Autodesk Fusion 360 part; units mm, degrees
(part 4 of 5)
  spline S1111 degree 3 poles (22.7215, 10.5636) (22.9807, 10.5636) (23.1283, 10.5984) (23.1913, 10.6743) knots 0 0 0 0 1 1 1 1
  spline S1112 degree 3 poles (-24.4021, 10.7683) (-24.3137, 10.8038) (-23.9421, 10.9498) (-23.5763, 11.0927) knots 0 0 0 0 1 1 1 1
  spline S1113 degree 3 poles (-23.5763, 11.0927) (-22.2598, 11.6068) (-21.6203, 11.9103) (-21.579, 12.0405) knots 0 0 0 0 1 1 1 1
  spline S1114 degree 3 poles (-21.579, 12.0405) (-21.5566, 12.1111) (-21.5714, 12.2881) (-21.6118, 12.4338) knots 0 0 0 0 1 1 1 1
  spline S1115 degree 3 poles (-21.6118, 12.4338) (-21.6523, 12.5796) (-21.6856, 12.7805) (-21.6858, 12.8804) knots 0 0 0 0 1 1 1 1
  spline S1116 degree 3 poles (-21.6858, 12.8804) (-21.686, 12.9803) (-21.7458, 13.116) (-21.8186, 13.1819) knots 0 0 0 0 1 1 1 1
  spline S1117 degree 3 poles (-21.8186, 13.1819) (-21.9416, 13.2933) (-22.0025, 13.2944) (-22.6762, 13.1972) knots 0 0 0 0 1 1 1 1
  spline S1118 degree 3 poles (-22.6762, 13.1972) (-23.075, 13.1397) (-23.7635, 13.0561) (-24.2063, 13.0113) knots 0 0 0 0 1 1 1 1
  spline S1119 degree 3 poles (-24.2063, 13.0113) (-24.6491, 12.9665) (-25.0546, 12.8945) (-25.1075, 12.8511) knots 0 0 0 0 1 1 1 1
  spline S1120 degree 3 poles (-25.1075, 12.8511) (-25.2214, 12.7577) (-25.1757, 12.0662) (-25.0076, 11.3415) knots 0 0 0 0 1 1 1 1
  spline S1121 degree 3 poles (-25.0076, 11.3415) (-24.8606, 10.7078) (-24.7688, 10.6209) (-24.4021, 10.7683) knots 0 0 0 0 1 1 1 1
  spline S1122 degree 3 poles (21.2509, 11.2698) (21.326, 11.377) (21.3366, 11.4739) (21.2907, 11.634) knots 0 0 0 0 1 1 1 1
  spline S1123 degree 3 poles (21.2907, 11.634) (21.1709, 12.0516) (21.2089, 12.044) (18.9436, 12.1086) knots 0 0 0 0 1 1 1 1
  spline S1124 degree 3 poles (18.9436, 12.1086) (17.0607, 12.1623) (16.8438, 12.157) (16.7302, 12.0542) knots 0 0 0 0 1 1 1 1
  spline S1125 degree 3 poles (16.7302, 12.0542) (16.6337, 11.9669) (16.6147, 11.8816) (16.6491, 11.6895) knots 0 0 0 0 1 1 1 1
  spline S1126 degree 3 poles (16.6491, 11.6895) (16.7375, 11.1953) (16.7258, 11.1985) (18.4885, 11.1761) knots 0 0 0 0 1 1 1 1
  spline S1127 degree 3 poles (18.4885, 11.1761) (19.3591, 11.165) (20.3138, 11.1487) (20.61, 11.1398) knots 0 0 0 0 1 1 1 1
  spline S1128 degree 3 poles (20.61, 11.1398) (21.0869, 11.1255) (21.1603, 11.1404) (21.2509, 11.2698) knots 0 0 0 0 1 1 1 1
  spline S1129 degree 3 poles (-19.2079, 11.7134) (-18.8576, 11.9992) (-18.3505, 12.4375) (-18.0809, 12.6873) knots 0 0 0 0 1 1 1 1
  spline S1130 degree 3 poles (-18.0809, 12.6873) (-17.6144, 13.1198) (-17.5967, 13.1475) (-17.7119, 13.2662) knots 0 0 0 0 1 1 1 1
  spline S1131 degree 3 poles (-17.7119, 13.2662) (-17.8279, 13.3856) (-17.8483, 13.3846) (-18.202, 13.2406) knots 0 0 0 0 1 1 1 1
  spline S1132 degree 3 poles (-18.202, 13.2406) (-19.0738, 12.8857) (-20.2187, 12.4538) (-20.2877, 12.4538) knots 0 0 0 0 1 1 1 1
  spline S1133 degree 3 poles (-20.2877, 12.4538) (-20.3288, 12.4538) (-20.4422, 12.374) (-20.5396, 12.2766) knots 0 0 0 0 1 1 1 1
  line L139 (-20.5396, 12.2766) -> (-20.7168, 12.0994)
  line L140 (-20.7168, 12.0994) -> (-20.5267, 11.769)
  spline S1134 degree 3 poles (-20.5267, 11.769) (-20.2684, 11.3201) (-20.1493, 11.1937) (-19.9846, 11.1937) knots 0 0 0 0 1 1 1 1
  spline S1135 degree 3 poles (-19.9846, 11.1937) (-19.9078, 11.1937) (-19.5583, 11.4275) (-19.2079, 11.7134) knots 0 0 0 0 1 1 1 1
  spline S1136 degree 3 poles (-13.2368, 11.7436) (-12.6043, 12.2729) (-12.0764, 12.8629) (-12.1241, 12.9872) knots 0 0 0 0 1 1 1 1
  spline S1137 degree 3 poles (-12.1241, 12.9872) (-12.1469, 13.0466) (-12.1656, 13.1242) (-12.1656, 13.1595) knots 0 0 0 0 1 1 1 1
  spline S1138 degree 3 poles (-12.1656, 13.1595) (-12.1656, 13.1949) (-12.1975, 13.2238) (-12.2366, 13.2238) knots 0 0 0 0 1 1 1 1
  spline S1139 degree 3 poles (-12.2366, 13.2238) (-12.2756, 13.2238) (-12.7001, 13.4012) (-13.1798, 13.6181) knots 0 0 0 0 1 1 1 1
  spline S1140 degree 3 poles (-13.1798, 13.6181) (-14.0327, 14.0036) (-14.0561, 14.0097) (-14.2327, 13.894) knots 0 0 0 0 1 1 1 1
  spline S1141 degree 3 poles (-14.2327, 13.894) (-14.332, 13.8289) (-14.4315, 13.7282) (-14.4538, 13.6701) knots 0 0 0 0 1 1 1 1
  spline S1142 degree 3 poles (-14.4538, 13.6701) (-14.512, 13.5184) (-13.9849, 11.5956) (-13.8565, 11.4912) knots 0 0 0 0 1 1 1 1
  spline S1143 degree 3 poles (-13.8565, 11.4912) (-13.6999, 11.3638) (-13.6817, 11.3712) (-13.2368, 11.7436) knots 0 0 0 0 1 1 1 1
  spline S1144 degree 3 poles (-8.9533, 13.0095) (-8.8858, 13.0457) (-8.7742, 13.2) (-8.7055, 13.3525) knots 0 0 0 0 1 1 1 1
  spline S1145 degree 3 poles (-8.7055, 13.3525) (-8.4998, 13.8087) (-8.5846, 13.8736) (-9.5179, 13.9744) knots 0 0 0 0 1 1 1 1
  line L141 (-9.5179, 13.9744) -> (-10.3105, 14.06)
  line L142 (-10.3105, 14.06) -> (-10.468, 13.883)
  spline S1146 degree 3 poles (-10.468, 13.883) (-10.7752, 13.5378) (-10.6837, 13.4311) (-9.8554, 13.1682) knots 0 0 0 0 1 1 1 1
  spline S1147 degree 3 poles (-9.8554, 13.1682) (-9.0718, 12.9194) (-9.1093, 12.926) (-8.9533, 13.0095) knots 0 0 0 0 1 1 1 1
  spline S1148 degree 3 poles (-18.991, 13.7481) (-18.7215, 13.8542) (-18.2394, 14.0518) (-17.9197, 14.1873) knots 0 0 0 0 1 1 1 1
  spline S1149 degree 3 poles (-17.9197, 14.1873) (-17.3857, 14.4137) (-17.3402, 14.4485) (-17.3597, 14.6163) knots 0 0 0 0 1 1 1 1
  line L143 (-17.3597, 14.6163) -> (-17.3809, 14.7989)
  line L144 (-17.3809, 14.7989) -> (-19.026, 14.8367)
  spline S1150 degree 3 poles (-19.026, 14.8367) (-21.0331, 14.8829) (-20.9284, 14.9282) (-20.9731, 13.9937) knots 0 0 0 0 1 1 1 1
  spline S1151 degree 3 poles (-20.9731, 13.9937) (-20.9985, 13.4622) (-20.9838, 13.3373) (-20.8825, 13.2253) knots 0 0 0 0 1 1 1 1
  spline S1152 degree 3 poles (-20.8825, 13.2253) (-20.7638, 13.0942) (-20.749, 13.0961) (-20.1212, 13.3234) knots 0 0 0 0 1 1 1 1
  spline S1153 degree 3 poles (-20.1212, 13.3234) (-19.7691, 13.4509) (-19.2605, 13.642) (-18.991, 13.7481) knots 0 0 0 0 1 1 1 1
  spline S1154 degree 3 poles (-23.3146, 13.8917) (-22.5289, 13.9927) (-21.893, 14.1075) (-21.8429, 14.1575) knots 0 0 0 0 1 1 1 1
  spline S1155 degree 3 poles (-21.8429, 14.1575) (-21.7944, 14.2058) (-21.7099, 14.4959) (-21.6552, 14.8022) knots 0 0 0 0 1 1 1 1
  spline S1156 degree 3 poles (-21.6552, 14.8022) (-21.6005, 15.1084) (-21.5059, 15.4981) (-21.4449, 15.6681) knots 0 0 0 0 1 1 1 1
  spline S1157 degree 3 poles (-21.4449, 15.6681) (-21.384, 15.8382) (-21.3519, 16.0334) (-21.3737, 16.1019) knots 0 0 0 0 1 1 1 1
  spline S1158 degree 3 poles (-21.3737, 16.1019) (-21.396, 16.1723) (-21.5793, 16.2891) (-21.7947, 16.3703) knots 0 0 0 0 1 1 1 1
  spline S1159 degree 3 poles (-21.7947, 16.3703) (-22.0045, 16.4493) (-22.3573, 16.5815) (-22.5787, 16.664) knots 0 0 0 0 1 1 1 1
  spline S1160 degree 3 poles (-22.5787, 16.664) (-22.8001, 16.7464) (-23.2138, 16.9206) (-23.4981, 17.0509) knots 0 0 0 0 1 1 1 1
  spline S1161 degree 3 poles (-23.4981, 17.0509) (-23.9693, 17.267) (-24.0287, 17.279) (-24.1702, 17.1862) knots 0 0 0 0 1 1 1 1
  spline S1162 degree 3 poles (-24.1702, 17.1862) (-24.5551, 16.9341) (-25.2902, 14.1127) (-25.0473, 13.82) knots 0 0 0 0 1 1 1 1
  spline S1163 degree 3 poles (-25.0473, 13.82) (-24.9336, 13.683) (-24.9403, 13.6827) (-23.3146, 13.8917) knots 0 0 0 0 1 1 1 1
  spline S1164 degree 3 poles (-11.5027, 13.8277) (-11.4398, 13.8518) (-11.2771, 14.0925) (-11.1411, 14.3625) knots 0 0 0 0 1 1 1 1
  spline S1165 degree 3 poles (-11.1411, 14.3625) (-10.902, 14.8374) (-10.8981, 14.8575) (-11.0222, 14.9768) knots 0 0 0 0 1 1 1 1
  spline S1166 degree 3 poles (-11.0222, 14.9768) (-11.1429, 15.0929) (-11.2111, 15.0941) (-12.1656, 14.9984) knots 0 0 0 0 1 1 1 1
  spline S1167 degree 3 poles (-12.1656, 14.9984) (-13.3577, 14.8788) (-13.3556, 14.8794) (-13.3556, 14.6979) knots 0 0 0 0 1 1 1 1
  spline S1168 degree 3 poles (-13.3556, 14.6979) (-13.3556, 14.5391) (-13.2065, 14.4507) (-12.2706, 14.0546) knots 0 0 0 0 1 1 1 1
  spline S1169 degree 3 poles (-12.2706, 14.0546) (-11.5304, 13.7413) (-11.6419, 13.7743) (-11.5027, 13.8277) knots 0 0 0 0 1 1 1 1
  spline S1170 degree 3 poles (-15.122, 14.2422) (-14.6101, 14.4561) (-14.2657, 14.9516) (-14.2657, 15.4741) knots 0 0 0 0 1 1 1 1
  spline S1171 degree 3 poles (-14.2657, 15.4741) (-14.2657, 15.8959) (-14.4671, 16.094) (-14.8959, 16.094) knots 0 0 0 0 1 1 1 1
  spline S1172 degree 3 poles (-14.8959, 16.094) (-15.8095, 16.094) (-16.5832, 14.8175) (-15.9994, 14.2736) knots 0 0 0 0 1 1 1 1
  spline S1173 degree 3 poles (-15.9994, 14.2736) (-15.8183, 14.1049) (-15.4797, 14.0927) (-15.122, 14.2422) knots 0 0 0 0 1 1 1 1
  spline S1174 degree 3 poles (-8.003, 14.785) (-7.8424, 15.0302) (-7.341, 16.6099) (-7.3194, 16.939) knots 0 0 0 0 1 1 1 1
  spline S1175 degree 3 poles (-7.3194, 16.939) (-7.2863, 17.4417) (-7.3904, 17.4406) (-8.5646, 16.9264) knots 0 0 0 0 1 1 1 1
  spline S1176 degree 3 poles (-8.5646, 16.9264) (-9.1332, 16.6774) (-9.6221, 16.4276) (-9.6509, 16.3713) knots 0 0 0 0 1 1 1 1
  spline S1177 degree 3 poles (-9.6509, 16.3713) (-9.6797, 16.3151) (-9.7716, 15.9734) (-9.8551, 15.6122) knots 0 0 0 0 1 1 1 1
  spline S1178 degree 3 poles (-9.8551, 15.6122) (-10.0402, 14.8114) (-10.0253, 14.7874) (-9.2924, 14.7025) knots 0 0 0 0 1 1 1 1
  spline S1179 degree 3 poles (-9.2924, 14.7025) (-8.3312, 14.5912) (-8.1212, 14.6046) (-8.003, 14.785) knots 0 0 0 0 1 1 1 1
  spline S1180 degree 3 poles (-17.7099, 15.6179) (-17.5251, 15.8028) (-17.6358, 15.9384) (-18.3085, 16.3507) knots 0 0 0 0 1 1 1 1
  spline S1181 degree 3 poles (-18.3085, 16.3507) (-18.6839, 16.5809) (-19.1537, 16.8723) (-19.3526, 16.9984) knots 0 0 0 0 1 1 1 1
  spline S1182 degree 3 poles (-19.3526, 16.9984) (-19.6303, 17.1744) (-19.7429, 17.2116) (-19.8376, 17.1586) knots 0 0 0 0 1 1 1 1
  spline S1183 degree 3 poles (-19.8376, 17.1586) (-19.9055, 17.1206) (-20.0957, 16.8262) (-20.2603, 16.5042) knots 0 0 0 0 1 1 1 1
  spline S1184 degree 3 poles (-20.2603, 16.5042) (-20.6962, 15.6518) (-20.6935, 15.6494) (-19.2276, 15.6013) knots 0 0 0 0 1 1 1 1
  spline S1185 degree 3 poles (-19.2276, 15.6013) (-18.597, 15.5806) (-18.0164, 15.557) (-17.9374, 15.5488) knots 0 0 0 0 1 1 1 1
  spline S1186 degree 3 poles (-17.9374, 15.5488) (-17.8585, 15.5406) (-17.7561, 15.5717) (-17.7099, 15.6179) knots 0 0 0 0 1 1 1 1
  spline S1187 degree 3 poles (-11.1991, 15.8565) (-10.6041, 15.9191) (-10.4912, 16.0246) (-10.4685, 16.5393) knots 0 0 0 0 1 1 1 1
  spline S1188 degree 3 poles (-10.4685, 16.5393) (-10.4402, 17.1834) (-10.5209, 17.1892) (-11.4906, 16.6128) knots 0 0 0 0 1 1 1 1
  spline S1189 degree 3 poles (-11.4906, 16.6128) (-12.1123, 16.2431) (-12.3045, 16.0946) (-12.305, 15.9831) knots 0 0 0 0 1 1 1 1
  spline S1190 degree 3 poles (-12.305, 15.9831) (-12.3058, 15.7689) (-12.2332, 15.7288) (-11.921, 15.7717) knots 0 0 0 0 1 1 1 1
  spline S1191 degree 3 poles (-11.921, 15.7717) (-11.7668, 15.7928) (-11.4419, 15.831) (-11.1991, 15.8565) knots 0 0 0 0 1 1 1 1
  spline S1192 degree 3 poles (-29.4487, 16.0958) (-29.2413, 16.1353) (-28.2608, 16.2435) (-27.2697, 16.3363) knots 0 0 0 0 1 1 1 1
  spline S1193 degree 3 poles (-27.2697, 16.3363) (-26.2787, 16.429) (-25.4399, 16.5221) (-25.4057, 16.5432) knots 0 0 0 0 1 1 1 1
  spline S1194 degree 3 poles (-25.4057, 16.5432) (-25.3716, 16.5643) (-25.2714, 16.7633) (-25.1832, 16.9853) knots 0 0 0 0 1 1 1 1
  spline S1195 degree 3 poles (-25.1832, 16.9853) (-24.9857, 17.4823) (-24.5021, 18.4625) (-24.2095, 18.9587) knots 0 0 0 0 1 1 1 1
  spline S1196 degree 3 poles (-24.2095, 18.9587) (-24.0275, 19.2675) (-24.0058, 19.3479) (-24.079, 19.444) knots 0 0 0 0 1 1 1 1
  spline S1197 degree 3 poles (-24.079, 19.444) (-24.1272, 19.5074) (-24.1706, 19.5673) (-24.1754, 19.5772) knots 0 0 0 0 1 1 1 1
  spline S1198 degree 3 poles (-24.1754, 19.5772) (-24.192, 19.6118) (-26.0679, 19.3801) (-26.9015, 19.2405) knots 0 0 0 0 1 1 1 1
  spline S1199 degree 3 poles (-26.9015, 19.2405) (-27.3635, 19.1631) (-27.932, 19.0374) (-28.1647, 18.9611) knots 0 0 0 0 1 1 1 1
  spline S1200 degree 3 poles (-28.1647, 18.9611) (-28.5842, 18.8235) (-28.5912, 18.8168) (-28.9823, 18.1757) knots 0 0 0 0 1 1 1 1
  spline S1201 degree 3 poles (-28.9823, 18.1757) (-29.1993, 17.82) (-29.5234, 17.2641) (-29.7025, 16.9402) knots 0 0 0 0 1 1 1 1
  spline S1202 degree 3 poles (-29.7025, 16.9402) (-29.9932, 16.4146) (-30.0188, 16.3337) (-29.9406, 16.1876) knots 0 0 0 0 1 1 1 1
  spline S1203 degree 3 poles (-29.9406, 16.1876) (-29.8924, 16.0976) (-29.8469, 16.024) (-29.8394, 16.024) knots 0 0 0 0 1 1 1 1
  spline S1204 degree 3 poles (-29.8394, 16.024) (-29.8319, 16.024) (-29.6561, 16.0563) (-29.4487, 16.0958) knots 0 0 0 0 1 1 1 1
  spline S1205 degree 3 poles (-16.2395, 16.4188) (-16.2187, 16.5646) (-16.4568, 17.3401) (-16.9745, 18.8132) knots 0 0 0 0 1 1 1 1
  spline S1206 degree 3 poles (-16.9745, 18.8132) (-17.2943, 19.723) (-17.3662, 19.7643) (-17.906, 19.3491) knots 0 0 0 0 1 1 1 1
  spline S1207 degree 3 poles (-17.906, 19.3491) (-18.4508, 18.93) (-19.236, 18.1166) (-19.236, 17.9714) knots 0 0 0 0 1 1 1 1
  spline S1208 degree 3 poles (-19.236, 17.9714) (-19.236, 17.848) (-18.823, 17.5592) (-17.3849, 16.6773) knots 0 0 0 0 1 1 1 1
  spline S1209 degree 3 poles (-17.3849, 16.6773) (-16.6183, 16.2071) (-16.2805, 16.1309) (-16.2395, 16.4188) knots 0 0 0 0 1 1 1 1
  spline S1210 degree 3 poles (24.6841, 16.7418) (24.7472, 16.8421) (24.6348, 17.1146) (24.0681, 18.2358) knots 0 0 0 0 1 1 1 1
  spline S1211 degree 3 poles (24.0681, 18.2358) (23.6075, 19.147) (23.3258, 19.6277) (23.2283, 19.6685) knots 0 0 0 0 1 1 1 1
  spline S1212 degree 3 poles (23.2283, 19.6685) (23.1476, 19.7022) (22.4538, 19.7782) (21.6865, 19.8372) knots 0 0 0 0 1 1 1 1
  spline S1213 degree 3 poles (21.6865, 19.8372) (20.7303, 19.9108) (20.2419, 19.977) (20.134, 20.0476) knots 0 0 0 0 1 1 1 1
  spline S1214 degree 3 poles (20.134, 20.0476) (20.0474, 20.1044) (19.797, 20.4587) (19.5775, 20.835) knots 0 0 0 0 1 1 1 1
  spline S1215 degree 3 poles (19.5775, 20.835) (19.358, 21.2114) (19.0588, 21.6802) (18.9126, 21.8768) knots 0 0 0 0 1 1 1 1
  line L145 (18.9126, 21.8768) -> (18.6469, 22.2344)
  line L146 (18.6469, 22.2344) -> (17.294, 22.3167)
  spline S1216 degree 3 poles (17.294, 22.3167) (16.55, 22.362) (15.8373, 22.412) (15.7104, 22.4278) knots 0 0 0 0 1 1 1 1
  spline S1217 degree 3 poles (15.7104, 22.4278) (15.5213, 22.4514) (15.4661, 22.427) (15.4048, 22.2924) knots 0 0 0 0 1 1 1 1
  spline S1218 degree 3 poles (15.4048, 22.2924) (15.3433, 22.1575) (15.3768, 22.007) (15.5924, 21.4507) knots 0 0 0 0 1 1 1 1
  line L147 (15.5924, 21.4507) -> (15.8549, 20.7732)
  line L148 (15.8549, 20.7732) -> (15.6497, 20.4812)
  line L149 (15.6497, 20.4812) -> (15.4444, 20.1892)
  line L150 (15.4444, 20.1892) -> (14.5027, 20.2093)
  spline S1219 degree 3 poles (14.5027, 20.2093) (13.9848, 20.2204) (13.2933, 20.2428) (12.966, 20.2592) knots 0 0 0 0 1 1 1 1
  spline S1220 degree 3 poles (12.966, 20.2592) (12.6387, 20.2755) (11.5034, 20.3093) (10.4432, 20.3342) knots 0 0 0 0 1 1 1 1
  spline S1221 degree 3 poles (10.4432, 20.3342) (8.7029, 20.375) (8.5061, 20.3681) (8.4196, 20.2639) knots 0 0 0 0 1 1 1 1
  spline S1222 degree 3 poles (8.4196, 20.2639) (8.3377, 20.1652) (8.3576, 19.9424) (8.556, 18.7337) knots 0 0 0 0 1 1 1 1
  spline S1223 degree 3 poles (8.556, 18.7337) (8.711, 17.7902) (8.8254, 17.2814) (8.8995, 17.206) knots 0 0 0 0 1 1 1 1
  spline S1224 degree 3 poles (8.8995, 17.206) (8.9972, 17.1068) (9.5698, 17.0787) (13.596, 16.9752) knots 0 0 0 0 1 1 1 1
  spline S1225 degree 3 poles (13.596, 16.9752) (18.7286, 16.8432) (19.6049, 16.8128) (21.8565, 16.6884) knots 0 0 0 0 1 1 1 1
  spline S1226 degree 3 poles (21.8565, 16.6884) (23.9806, 16.5711) (24.5839, 16.5825) (24.6841, 16.7418) knots 0 0 0 0 1 1 1 1
  spline S1227 degree 3 poles (-11.963, 17.225) (-11.6316, 17.4236) (-11.1758, 17.7107) (-10.9501, 17.863) knots 0 0 0 0 1 1 1 1
  spline S1228 degree 3 poles (-10.9501, 17.863) (-10.5619, 18.1251) (-10.5418, 18.1526) (-10.5777, 18.3738) knots 0 0 0 0 1 1 1 1
  spline S1229 degree 3 poles (-10.5777, 18.3738) (-10.6459, 18.794) (-10.9302, 19.2768) (-11.123, 19.2999) knots 0 0 0 0 1 1 1 1
  spline S1230 degree 3 poles (-11.123, 19.2999) (-11.2688, 19.3174) (-11.3514, 19.2395) (-11.6426, 18.8099) knots 0 0 0 0 1 1 1 1
  spline S1231 degree 3 poles (-11.6426, 18.8099) (-11.833, 18.529) (-12.1895, 18.0229) (-12.4348, 17.6853) knots 0 0 0 0 1 1 1 1
  spline S1232 degree 3 poles (-12.4348, 17.6853) (-12.8031, 17.1783) (-12.8657, 17.0535) (-12.7946, 16.9678) knots 0 0 0 0 1 1 1 1
  spline S1233 degree 3 poles (-12.7946, 16.9678) (-12.7472, 16.9107) (-12.6763, 16.864) (-12.637, 16.864) knots 0 0 0 0 1 1 1 1
  spline S1234 degree 3 poles (-12.637, 16.864) (-12.5977, 16.864) (-12.2944, 17.0265) (-11.963, 17.225) knots 0 0 0 0 1 1 1 1
  spline S1235 degree 3 poles (-20.8903, 17.0639) (-20.8256, 17.1354) (-20.7917, 17.2431) (-20.8148, 17.3034) knots 0 0 0 0 1 1 1 1
  spline S1236 degree 3 poles (-20.8148, 17.3034) (-20.8533, 17.4038) (-22.872, 18.7732) (-23.1241, 18.8699) knots 0 0 0 0 1 1 1 1
  spline S1237 degree 3 poles (-23.1241, 18.8699) (-23.3444, 18.9545) (-23.7875, 18.3407) (-23.6899, 18.0863) knots 0 0 0 0 1 1 1 1
  spline S1238 degree 3 poles (-23.6899, 18.0863) (-23.6666, 18.0255) (-23.4346, 17.8783) (-23.1744, 17.7589) knots 0 0 0 0 1 1 1 1
  spline S1239 degree 3 poles (-23.1744, 17.7589) (-22.5961, 17.4938) (-21.1899, 16.9406) (-21.0845, 16.9368) knots 0 0 0 0 1 1 1 1
  spline S1240 degree 3 poles (-21.0845, 16.9368) (-21.0423, 16.9353) (-20.9549, 16.9925) (-20.8903, 17.0639) knots 0 0 0 0 1 1 1 1
  spline S1241 degree 3 poles (-1.9745, 17.2186) (-1.9197, 17.264) (-1.876, 17.729) (-1.8449, 18.5982) knots 0 0 0 0 1 1 1 1
  spline S1242 degree 3 poles (-1.8449, 18.5982) (-1.7806, 20.3917) (-1.6759, 22.7737) (-1.624, 23.6226) knots 0 0 0 0 1 1 1 1
  spline S1243 degree 3 poles (-1.624, 23.6226) (-1.5882, 24.2076) (-1.5991, 24.3408) (-1.6891, 24.4155) knots 0 0 0 0 1 1 1 1
  spline S1244 degree 3 poles (-1.6891, 24.4155) (-1.8113, 24.5169) (-3.3464, 24.5276) (-6.4842, 24.4489) knots 0 0 0 0 1 1 1 1
  spline S1245 degree 3 poles (-6.4842, 24.4489) (-8.3278, 24.4026) (-8.3283, 24.4025) (-8.4027, 24.2393) knots 0 0 0 0 1 1 1 1
  spline S1246 degree 3 poles (-8.4027, 24.2393) (-8.4687, 24.0945) (-8.4379, 24.0343) (-8.1304, 23.7077) knots 0 0 0 0 1 1 1 1
  spline S1247 degree 3 poles (-8.1304, 23.7077) (-6.8687, 22.3676) (-6.2732, 20.5027) (-6.3844, 18.2404) knots 0 0 0 0 1 1 1 1
  spline S1248 degree 3 poles (-6.3844, 18.2404) (-6.4135, 17.6483) (-6.4058, 17.24) (-6.3646, 17.1903) knots 0 0 0 0 1 1 1 1
  spline S1249 degree 3 poles (-6.3646, 17.1903) (-6.2792, 17.0872) (-2.1003, 17.1142) (-1.9745, 17.2186) knots 0 0 0 0 1 1 1 1
  spline S1250 degree 3 poles (7.9228, 17.1756) (8.0336, 17.3091) (7.9974, 17.6663) (7.7218, 19.1614) knots 0 0 0 0 1 1 1 1
  spline S1251 degree 3 poles (7.7218, 19.1614) (7.6131, 19.7512) (7.487, 20.2709) (7.4414, 20.3165) knots 0 0 0 0 1 1 1 1
  spline S1252 degree 3 poles (7.4414, 20.3165) (7.3827, 20.3753) (6.7665, 20.406) (5.3145, 20.4227) knots 0 0 0 0 1 1 1 1
  line L151 (5.3145, 20.4227) -> (3.2704, 20.4461)
  line L152 (3.2704, 20.4461) -> (3.048, 20.6589)
  spline S1253 degree 3 poles (3.048, 20.6589) (2.8474, 20.8509) (2.8214, 20.924) (2.7826, 21.4055) knots 0 0 0 0 1 1 1 1
  spline S1254 degree 3 poles (2.7826, 21.4055) (2.662, 22.8997) (2.5206, 24.1965) (2.4629, 24.337) knots 0 0 0 0 1 1 1 1
  spline S1255 degree 3 poles (2.4629, 24.337) (2.3987, 24.4936) (2.3893, 24.4945) (0.8653, 24.4945) knots 0 0 0 0 1 1 1 1
  spline S1256 degree 3 poles (0.8653, 24.4945) (-0.4157, 24.4945) (-0.6821, 24.4771) (-0.7554, 24.3889) knots 0 0 0 0 1 1 1 1
  spline S1257 degree 3 poles (-0.7554, 24.3889) (-0.8521, 24.2723) (-0.9043, 23.4082) (-1.0395, 19.6829) knots 0 0 0 0 1 1 1 1
  spline S1258 degree 3 poles (-1.0395, 19.6829) (-1.107, 17.8242) (-1.1064, 17.3352) (-1.0364, 17.2509) knots 0 0 0 0 1 1 1 1
  spline S1259 degree 3 poles (-1.0364, 17.2509) (-0.961, 17.16) (-0.4774, 17.1428) (2.4559, 17.1272) knots 0 0 0 0 1 1 1 1
  spline S1260 degree 3 poles (2.4559, 17.1272) (4.3284, 17.1172) (6.3041, 17.0994) (6.8462, 17.0876) knots 0 0 0 0 1 1 1 1
  spline S1261 degree 3 poles (6.8462, 17.0876) (7.6728, 17.0696) (7.8466, 17.0838) (7.9228, 17.1756) knots 0 0 0 0 1 1 1 1
  spline S1262 degree 3 poles (-8.3794, 17.8468) (-7.0575, 18.4432) (-7.1146, 18.394) (-7.1395, 18.9154) knots 0 0 0 0 1 1 1 1
  spline S1263 degree 3 poles (-7.1395, 18.9154) (-7.1578, 19.2983) (-7.1779, 19.3517) (-7.3109, 19.3706) knots 0 0 0 0 1 1 1 1
  spline S1264 degree 3 poles (-7.3109, 19.3706) (-7.483, 19.3952) (-9.6454, 17.83) (-9.6454, 17.6809) knots 0 0 0 0 1 1 1 1
  spline S1265 degree 3 poles (-9.6454, 17.6809) (-9.6454, 17.5701) (-9.5041, 17.4241) (-9.3968, 17.4241) knots 0 0 0 0 1 1 1 1
  spline S1266 degree 3 poles (-9.3968, 17.4241) (-9.3525, 17.4241) (-8.8947, 17.6143) (-8.3794, 17.8468) knots 0 0 0 0 1 1 1 1
  spline S1267 degree 3 poles (-15.3671, 18.053) (-15.3369, 18.2641) (-15.3209, 18.8907) (-15.3315, 19.4455) knots 0 0 0 0 1 1 1 1
  spline S1268 degree 3 poles (-15.3315, 19.4455) (-15.3551, 20.6788) (-15.3656, 20.6931) (-16.0392, 20.4068) knots 0 0 0 0 1 1 1 1
  spline S1269 degree 3 poles (-16.0392, 20.4068) (-16.29, 20.3002) (-16.5129, 20.1668) (-16.5346, 20.1103) knots 0 0 0 0 1 1 1 1
  spline S1270 degree 3 poles (-16.5346, 20.1103) (-16.5563, 20.0538) (-16.3933, 19.4725) (-16.1724, 18.8184) knots 0 0 0 0 1 1 1 1
  spline S1271 degree 3 poles (-16.1724, 18.8184) (-15.7888, 17.6826) (-15.763, 17.6302) (-15.5964, 17.6492) knots 0 0 0 0 1 1 1 1
  spline S1272 degree 3 poles (-15.5964, 17.6492) (-15.4421, 17.6668) (-15.4157, 17.7133) (-15.3671, 18.053) knots 0 0 0 0 1 1 1 1
  spline S1273 degree 3 poles (-19.9804, 18.3806) (-19.8405, 18.5602) (-19.726, 18.7507) (-19.726, 18.804) knots 0 0 0 0 1 1 1 1
  spline S1274 degree 3 poles (-19.726, 18.804) (-19.726, 18.8573) (-19.9944, 19.2023) (-20.3223, 19.5707) knots 0 0 0 0 1 1 1 1
  spline S1275 degree 3 poles (-20.3223, 19.5707) (-20.6503, 19.939) (-21.0362, 20.3929) (-21.1799, 20.5794) knots 0 0 0 0 1 1 1 1
  spline S1276 degree 3 poles (-21.1799, 20.5794) (-21.5341, 21.039) (-21.6932, 21.0349) (-22.1105, 20.5559) knots 0 0 0 0 1 1 1 1
  spline S1277 degree 3 poles (-22.1105, 20.5559) (-22.6039, 19.9894) (-22.7587, 19.7538) (-22.7141, 19.6374) knots 0 0 0 0 1 1 1 1
  spline S1278 degree 3 poles (-22.7141, 19.6374) (-22.6624, 19.5027) (-20.501, 18.0579) (-20.3479, 18.0557) knots 0 0 0 0 1 1 1 1
  spline S1279 degree 3 poles (-20.3479, 18.0557) (-20.2857, 18.0548) (-20.1203, 18.201) (-19.9804, 18.3806) knots 0 0 0 0 1 1 1 1
  spline S1280 degree 3 poles (-13.8919, 18.9349) (-13.7055, 19.3937) (-13.4904, 19.9226) (-13.4138, 20.11) knots 0 0 0 0 1 1 1 1
  spline S1281 degree 3 poles (-13.4138, 20.11) (-13.1823, 20.6768) (-13.3092, 20.8511) (-13.9548, 20.8533) knots 0 0 0 0 1 1 1 1
  spline S1282 degree 3 poles (-13.9548, 20.8533) (-14.4887, 20.8551) (-14.5056, 20.8149) (-14.5498, 19.4425) knots 0 0 0 0 1 1 1 1
  spline S1283 degree 3 poles (-14.5498, 19.4425) (-14.583, 18.4103) (-14.573, 18.2159) (-14.4826, 18.1407) knots 0 0 0 0 1 1 1 1
  spline S1284 degree 3 poles (-14.4826, 18.1407) (-14.4242, 18.092) (-14.3436, 18.0631) (-14.3035, 18.0764) knots 0 0 0 0 1 1 1 1
  spline S1285 degree 3 poles (-14.3035, 18.0764) (-14.2635, 18.0896) (-14.0782, 18.476) (-13.8919, 18.9349) knots 0 0 0 0 1 1 1 1
  spline S1286 degree 3 poles (-12.3167, 19.2004) (-11.7607, 20.0152) (-11.7206, 20.1966) (-12.0622, 20.3522) knots 0 0 0 0 1 1 1 1
  spline S1287 degree 3 poles (-12.0622, 20.3522) (-12.4177, 20.5142) (-12.4624, 20.4628) (-12.8606, 19.432) knots 0 0 0 0 1 1 1 1
  spline S1288 degree 3 poles (-12.8606, 19.432) (-13.1686, 18.635) (-13.1918, 18.5374) (-13.0871, 18.4765) knots 0 0 0 0 1 1 1 1
  spline S1289 degree 3 poles (-13.0871, 18.4765) (-13.0231, 18.4392) (-12.9391, 18.4173) (-12.9006, 18.4279) knots 0 0 0 0 1 1 1 1
  spline S1290 degree 3 poles (-12.9006, 18.4279) (-12.8621, 18.4385) (-12.5993, 18.7861) (-12.3167, 19.2004) knots 0 0 0 0 1 1 1 1
  spline S1291 degree 3 poles (-8.7354, 19.4121) (-8.2541, 19.7731) (-7.7347, 20.1784) (-7.5812, 20.3126) knots 0 0 0 0 1 1 1 1
  line L153 (-7.5812, 20.3126) -> (-7.3021, 20.5567)
  line L154 (-7.3021, 20.5567) -> (-7.4675, 21.073)
  spline S1292 degree 3 poles (-7.4675, 21.073) (-7.7543, 21.9682) (-8.1644, 22.664) (-8.793, 23.3219) knots 0 0 0 0 1 1 1 1
  spline S1293 degree 3 poles (-8.793, 23.3219) (-9.0651, 23.6067) (-9.3183, 23.6618) (-9.437, 23.4619) knots 0 0 0 0 1 1 1 1
  spline S1294 degree 3 poles (-9.437, 23.4619) (-9.477, 23.3946) (-9.8553, 22.7592) (-10.2776, 22.0501) knots 0 0 0 0 1 1 1 1
  spline S1295 degree 3 poles (-10.2776, 22.0501) (-10.7, 21.3409) (-11.0455, 20.7206) (-11.0455, 20.6715) knots 0 0 0 0 1 1 1 1
  spline S1296 degree 3 poles (-11.0455, 20.6715) (-11.0455, 20.6225) (-10.8868, 20.401) (-10.6927, 20.1793) knots 0 0 0 0 1 1 1 1
  spline S1297 degree 3 poles (-10.6927, 20.1793) (-10.4987, 19.9576) (-10.2388, 19.5636) (-10.1152, 19.3038) knots 0 0 0 0 1 1 1 1
  spline S1298 degree 3 poles (-10.1152, 19.3038) (-9.9211, 18.8958) (-9.8416, 18.8044) (-9.6454, 18.763) knots 0 0 0 0 1 1 1 1
  spline S1299 degree 3 poles (-9.6454, 18.763) (-9.6262, 18.7589) (-9.2166, 19.051) (-8.7354, 19.4121) knots 0 0 0 0 1 1 1 1
  spline S1300 degree 3 poles (-18.6774, 19.7262) (-18.5, 19.8758) (-18.1042, 20.1617) (-17.7979, 20.3616) knots 0 0 0 0 1 1 1 1
  spline S1301 degree 3 poles (-17.7979, 20.3616) (-17.4915, 20.5615) (-17.2154, 20.7704) (-17.1842, 20.8259) knots 0 0 0 0 1 1 1 1
  spline S1302 degree 3 poles (-17.1842, 20.8259) (-17.1495, 20.8878) (-17.2127, 21.1625) (-17.3482, 21.538) knots 0 0 0 0 1 1 1 1
  spline S1303 degree 3 poles (-17.3482, 21.538) (-18.0947, 23.607) (-18.1162, 23.6544) (-18.3045, 23.6544) knots 0 0 0 0 1 1 1 1
  spline S1304 degree 3 poles (-18.3045, 23.6544) (-18.5773, 23.6544) (-20.8683, 21.9553) (-20.9523, 21.6907) knots 0 0 0 0 1 1 1 1
  spline S1305 degree 3 poles (-20.9523, 21.6907) (-20.9864, 21.5831) (-20.8624, 21.3906) (-20.4233, 20.8697) knots 0 0 0 0 1 1 1 1
  spline S1306 degree 3 poles (-20.4233, 20.8697) (-19.6725, 19.9791) (-19.1734, 19.4542) (-19.0774, 19.4542) knots 0 0 0 0 1 1 1 1
  spline S1307 degree 3 poles (-19.0774, 19.4542) (-19.0348, 19.4542) (-18.8549, 19.5766) (-18.6774, 19.7262) knots 0 0 0 0 1 1 1 1
  spline S1308 degree 3 poles (-26.5059, 20.0801) (-25.9919, 20.1548) (-25.0412, 20.2701) (-24.3931, 20.3362) knots 0 0 0 0 1 1 1 1
  line L155 (-24.3931, 20.3362) -> (-23.2148, 20.4564)
  line L156 (-23.2148, 20.4564) -> (-22.6367, 21.1279)
  spline S1309 degree 3 poles (-22.6367, 21.1279) (-22.0912, 21.7614) (-21.3699, 22.4498) (-20.6186, 23.0539) knots 0 0 0 0 1 1 1 1
  spline S1310 degree 3 poles (-20.6186, 23.0539) (-20.2532, 23.3478) (-20.2458, 23.3626) (-20.3762, 23.541) knots 0 0 0 0 1 1 1 1
  spline S1311 degree 3 poles (-20.3762, 23.541) (-20.4621, 23.6584) (-20.5191, 23.6573) (-21.5838, 23.5168) knots 0 0 0 0 1 1 1 1
  spline S1312 degree 3 poles (-21.5838, 23.5168) (-23.541, 23.2586) (-25.0365, 22.9504) (-25.5728, 22.6946) knots 0 0 0 0 1 1 1 1
  spline S1313 degree 3 poles (-25.5728, 22.6946) (-25.8037, 22.5845) (-26.5437, 21.7215) (-27.3461, 20.6266) knots 0 0 0 0 1 1 1 1
  spline S1314 degree 3 poles (-27.3461, 20.6266) (-27.5925, 20.2904) (-27.6289, 20.2007) (-27.5664, 20.084) knots 0 0 0 0 1 1 1 1
  spline S1315 degree 3 poles (-27.5664, 20.084) (-27.5253, 20.0071) (-27.4801, 19.9442) (-27.466, 19.9442) knots 0 0 0 0 1 1 1 1
  spline S1316 degree 3 poles (-27.466, 19.9442) (-27.4519, 19.9442) (-27.0199, 20.0054) (-26.5059, 20.0801) knots 0 0 0 0 1 1 1 1
  spline S1317 degree 3 poles (14.7535, 21.067) (14.8798, 21.2065) (14.8763, 21.2252) (14.5982, 21.9084) knots 0 0 0 0 1 1 1 1
  line L157 (14.5982, 21.9084) -> (14.3138, 22.6071)
  line L158 (14.3138, 22.6071) -> (14.5181, 22.9155)
  line L159 (14.5181, 22.9155) -> (14.7224, 23.2239)
  line L160 (14.7224, 23.2239) -> (15.6253, 23.1838)
  line L161 (15.6253, 23.1838) -> (16.5283, 23.1436)
  line L162 (16.5283, 23.1436) -> (16.5724, 23.3191)
  spline S1318 degree 3 poles (16.5724, 23.3191) (16.6067, 23.456) (16.5202, 23.6518) (16.1797, 24.2083) knots 0 0 0 0 1 1 1 1
  spline S1319 degree 3 poles (16.1797, 24.2083) (15.9395, 24.6008) (15.6893, 24.9507) (15.6237, 24.9858) knots 0 0 0 0 1 1 1 1
  spline S1320 degree 3 poles (15.6237, 24.9858) (15.5019, 25.051) (13.7255, 25.2193) (12.2495, 25.3055) knots 0 0 0 0 1 1 1 1
  spline S1321 degree 3 poles (12.2495, 25.3055) (11.3803, 25.3562) (11.2159, 25.3153) (11.2159, 25.048) knots 0 0 0 0 1 1 1 1
  spline S1322 degree 3 poles (11.2159, 25.048) (11.2159, 24.9768) (11.121, 24.7838) (11.0049, 24.6191) knots 0 0 0 0 1 1 1 1
  line L163 (11.0049, 24.6191) -> (10.794, 24.3195)
  line L164 (10.794, 24.3195) -> (9.9146, 24.3545)
  spline S1323 degree 3 poles (9.9146, 24.3545) (8.7135, 24.4023) (8.735, 24.4304) (9.0699, 23.2529) knots 0 0 0 0 1 1 1 1
  spline S1324 degree 3 poles (9.0699, 23.2529) (9.2097, 22.7615) (9.3891, 22.1074) (9.4686, 21.7993) knots 0 0 0 0 1 1 1 1
  spline S1325 degree 3 poles (9.4686, 21.7993) (9.5481, 21.4913) (9.6648, 21.1999) (9.7279, 21.1518) knots 0 0 0 0 1 1 1 1
  spline S1326 degree 3 poles (9.7279, 21.1518) (9.8066, 21.0917) (10.173, 21.0616) (10.8967, 21.0558) knots 0 0 0 0 1 1 1 1
  spline S1327 degree 3 poles (10.8967, 21.0558) (11.8311, 21.0482) (14.2155, 20.9697) (14.5127, 20.9367) knots 0 0 0 0 1 1 1 1
  spline S1328 degree 3 poles (14.5127, 20.9367) (14.5741, 20.9299) (14.6825, 20.9885) (14.7535, 21.067) knots 0 0 0 0 1 1 1 1
  spline S1329 degree 3 poles (-11.6859, 21.2639) (-11.5757, 21.3741) (-10.3192, 23.4398) (-10.0721, 23.917) knots 0 0 0 0 1 1 1 1
  spline S1330 degree 3 poles (-10.0721, 23.917) (-9.9126, 24.225) (-10.1886, 24.4387) (-11.175, 24.771) knots 0 0 0 0 1 1 1 1
  spline S1331 degree 3 poles (-11.175, 24.771) (-11.671, 24.9381) (-11.9074, 24.9519) (-12.0167, 24.8202) knots 0 0 0 0 1 1 1 1
  spline S1332 degree 3 poles (-12.0167, 24.8202) (-12.0598, 24.7682) (-12.1436, 24.4454) (-12.2029, 24.1026) knots 0 0 0 0 1 1 1 1
  spline S1333 degree 3 poles (-12.2029, 24.1026) (-12.2621, 23.7599) (-12.3895, 23.1329) (-12.4858, 22.7094) knots 0 0 0 0 1 1 1 1
  spline S1334 degree 3 poles (-12.4858, 22.7094) (-12.7304, 21.6341) (-12.736, 21.5988) (-12.675, 21.5112) knots 0 0 0 0 1 1 1 1
  spline S1335 degree 3 poles (-12.675, 21.5112) (-12.615, 21.4251) (-12.0417, 21.1495) (-11.9031, 21.1402) knots 0 0 0 0 1 1 1 1
  spline S1336 degree 3 poles (-11.9031, 21.1402) (-11.8549, 21.1369) (-11.7572, 21.1926) (-11.6859, 21.2639) knots 0 0 0 0 1 1 1 1
  spline S1337 degree 3 poles (5.6455, 21.2443) (5.7815, 21.3803) (5.7816, 21.4338) (5.6471, 22.1789) knots 0 0 0 0 1 1 1 1
  spline S1338 degree 3 poles (5.6471, 22.1789) (5.3745, 23.69) (5.2437, 24.2585) (5.1427, 24.372) knots 0 0 0 0 1 1 1 1
  spline S1339 degree 3 poles (5.1427, 24.372) (5.0512, 24.4749) (4.9082, 24.4945) (4.2504, 24.4945) knots 0 0 0 0 1 1 1 1
  spline S1340 degree 3 poles (4.2504, 24.4945) (3.5901, 24.4945) (3.4509, 24.4753) (3.3645, 24.372) knots 0 0 0 0 1 1 1 1
  spline S1341 degree 3 poles (3.3645, 24.372) (3.2742, 24.2641) (3.2792, 24.0763) (3.4061, 22.8004) knots 0 0 0 0 1 1 1 1
  spline S1342 degree 3 poles (3.4061, 22.8004) (3.4855, 22.0034) (3.5824, 21.3192) (3.6216, 21.2801) knots 0 0 0 0 1 1 1 1
  spline S1343 degree 3 poles (3.6216, 21.2801) (3.6607, 21.2409) (4.086, 21.1989) (4.5666, 21.1867) knots 0 0 0 0 1 1 1 1
  spline S1344 degree 3 poles (4.5666, 21.1867) (5.0472, 21.1745) (5.4618, 21.1578) (5.488, 21.1494) knots 0 0 0 0 1 1 1 1
  spline S1345 degree 3 poles (5.488, 21.1494) (5.5141, 21.1411) (5.585, 21.1838) (5.6455, 21.2443) knots 0 0 0 0 1 1 1 1
  line L165 (5.6455, 21.2443) -> (5.6455, 21.2443)
  spline S1346 degree 3 poles (8.7017, 21.2465) (8.7801, 21.3409) (8.7689, 21.4606) (8.6316, 21.9991) knots 0 0 0 0 1 1 1 1
  spline S1347 degree 3 poles (8.6316, 21.9991) (8.3635, 23.0501) (7.9905, 24.2438) (7.9027, 24.3314) knots 0 0 0 0 1 1 1 1
  spline S1348 degree 3 poles (7.9027, 24.3314) (7.8528, 24.3813) (7.5133, 24.4218) (7.0343, 24.4351) knots 0 0 0 0 1 1 1 1
  spline S1349 degree 3 poles (7.0343, 24.4351) (6.0604, 24.462) (5.9769, 24.4134) (6.0943, 23.8884) knots 0 0 0 0 1 1 1 1
  spline S1350 degree 3 poles (6.0943, 23.8884) (6.1812, 23.5004) (6.425, 22.1624) (6.4943, 21.6943) knots 0 0 0 0 1 1 1 1
  spline S1351 degree 3 poles (6.4943, 21.6943) (6.5735, 21.1582) (6.6242, 21.1343) (7.6829, 21.1343) knots 0 0 0 0 1 1 1 1
  spline S1352 degree 3 poles (7.6829, 21.1343) (8.4468, 21.1343) (8.6249, 21.1539) (8.7017, 21.2465) knots 0 0 0 0 1 1 1 1
  line L166 (-15.7008, 21.3381) -> (-15.3508, 21.461)
  line L167 (-15.3508, 21.461) -> (-15.328, 22.0502)
  spline S1353 degree 3 poles (-15.328, 22.0502) (-15.287, 23.1093) (-15.3862, 24.4796) (-15.5155, 24.6389) knots 0 0 0 0 1 1 1 1
  line L168 (-15.5155, 24.6389) -> (-15.6308, 24.781)
  line L169 (-15.6308, 24.781) -> (-16.0955, 24.6373)
  spline S1354 degree 3 poles (-16.0955, 24.6373) (-16.7706, 24.4286) (-17.3206, 24.1714) (-17.3706, 24.0409) knots 0 0 0 0 1 1 1 1
  spline S1355 degree 3 poles (-17.3706, 24.0409) (-17.3946, 23.9784) (-17.3081, 23.6532) (-17.1784, 23.3183) knots 0 0 0 0 1 1 1 1
  spline S1356 degree 3 poles (-17.1784, 23.3183) (-17.0486, 22.9834) (-16.8565, 22.4574) (-16.7515, 22.1493) knots 0 0 0 0 1 1 1 1
  spline S1357 degree 3 poles (-16.7515, 22.1493) (-16.4001, 21.1188) (-16.3767, 21.1007) (-15.7008, 21.3381) knots 0 0 0 0 1 1 1 1
  spline S1358 degree 3 poles (-13.6196, 21.6631) (-13.4863, 21.7404) (-13.329, 22.3099) (-13.0438, 23.7476) knots 0 0 0 0 1 1 1 1
  spline S1359 degree 3 poles (-13.0438, 23.7476) (-12.8309, 24.8207) (-12.8294, 24.8601) (-12.9955, 25.0104) knots 0 0 0 0 1 1 1 1
  spline S1360 degree 3 poles (-12.9955, 25.0104) (-13.1092, 25.1133) (-13.2105, 25.1201) (-13.8065, 25.0653) knots 0 0 0 0 1 1 1 1
  spline S1361 degree 3 poles (-13.8065, 25.0653) (-14.2477, 25.0248) (-14.5245, 24.9658) (-14.5925, 24.8977) knots 0 0 0 0 1 1 1 1
  spline S1362 degree 3 poles (-14.5925, 24.8977) (-14.683, 24.8072) (-14.687, 24.6702) (-14.6216, 23.9048) knots 0 0 0 0 1 1 1 1
  spline S1363 degree 3 poles (-14.6216, 23.9048) (-14.5799, 23.4164) (-14.5457, 22.7368) (-14.5457, 22.3945) knots 0 0 0 0 1 1 1 1
  spline S1364 degree 3 poles (-14.5457, 22.3945) (-14.5457, 21.8527) (-14.5277, 21.7596) (-14.4065, 21.6747) knots 0 0 0 0 1 1 1 1
  spline S1365 degree 3 poles (-14.4065, 21.6747) (-14.2488, 21.5643) (-13.8017, 21.5577) (-13.6196, 21.6631) knots 0 0 0 0 1 1 1 1
  spline S1366 degree 3 poles (-23.1212, 24.0714) (-22.6592, 24.1467) (-21.7142, 24.2729) (-21.0211, 24.3518) knots 0 0 0 0 1 1 1 1
  spline S1367 degree 3 poles (-21.0211, 24.3518) (-20.3281, 24.4307) (-19.6592, 24.5121) (-19.5346, 24.5328) knots 0 0 0 0 1 1 1 1
  spline S1368 degree 3 poles (-19.5346, 24.5328) (-19.3464, 24.5641) (-19.196, 24.7113) (-18.6419, 25.407) knots 0 0 0 0 1 1 1 1
  spline S1369 degree 3 poles (-18.6419, 25.407) (-17.0777, 27.3707) (-15.2803, 29.1546) (-13.5132, 30.4969) knots 0 0 0 0 1 1 1 1
  spline S1370 degree 3 poles (-13.5132, 30.4969) (-13.08, 30.8259) (-12.7256, 31.134) (-12.7256, 31.1814) knots 0 0 0 0 1 1 1 1
  spline S1371 degree 3 poles (-12.7256, 31.1814) (-12.7256, 31.2289) (-12.7708, 31.3052) (-12.8259, 31.351) knots 0 0 0 0 1 1 1 1
  spline S1372 degree 3 poles (-12.8259, 31.351) (-12.9051, 31.4167) (-13.1577, 31.374) (-14.023, 31.1487) knots 0 0 0 0 1 1 1 1
  spline S1373 degree 3 poles (-14.023, 31.1487) (-15.3494, 30.8033) (-15.8761, 30.59) (-17.0056, 29.941) knots 0 0 0 0 1 1 1 1
  spline S1374 degree 3 poles (-17.0056, 29.941) (-19.1855, 28.6885) (-21.5007, 26.9447) (-23.3488, 25.1635) knots 0 0 0 0 1 1 1 1
  spline S1375 degree 3 poles (-23.3488, 25.1635) (-24.1925, 24.3503) (-24.366, 24.1175) (-24.2296, 23.9811) knots 0 0 0 0 1 1 1 1
  spline S1376 degree 3 poles (-24.2296, 23.9811) (-24.1603, 23.9118) (-24.0412, 23.9215) (-23.1212, 24.0714) knots 0 0 0 0 1 1 1 1
  spline S1377 degree 3 poles (-17.0386, 25.1171) (-15.7226, 25.6239) (-14.4425, 25.8456) (-12.9706, 25.8216) knots 0 0 0 0 1 1 1 1
  spline S1378 degree 3 poles (-12.9706, 25.8216) (-12.4316, 25.8128) (-11.9551, 25.8099) (-11.9118, 25.8151) knots 0 0 0 0 1 1 1 1
  spline S1379 degree 3 poles (-11.9118, 25.8151) (-11.8684, 25.8203) (-11.6354, 26.179) (-11.394, 26.6121) knots 0 0 0 0 1 1 1 1
  spline S1380 degree 3 poles (-11.394, 26.6121) (-10.3842, 28.4235) (-9.2894, 29.9181) (-7.7957, 31.5245) knots 0 0 0 0 1 1 1 1
  spline S1381 degree 3 poles (-7.7957, 31.5245) (-7.4407, 31.9063) (-7.4389, 31.9107) (-7.5628, 32.0723) knots 0 0 0 0 1 1 1 1
  spline S1382 degree 3 poles (-7.5628, 32.0723) (-7.6436, 32.1777) (-7.7368, 32.1766) (-8.7773, 32.0579) knots 0 0 0 0 1 1 1 1
  spline S1383 degree 3 poles (-8.7773, 32.0579) (-10.014, 31.917) (-9.999, 31.9223) (-11.1155, 31.2288) knots 0 0 0 0 1 1 1 1
  spline S1384 degree 3 poles (-11.1155, 31.2288) (-12.6968, 30.2467) (-14.7654, 28.5663) (-16.0252, 27.2406) knots 0 0 0 0 1 1 1 1
  spline S1385 degree 3 poles (-16.0252, 27.2406) (-16.8136, 26.4108) (-17.8359, 25.2288) (-17.8359, 25.1469) knots 0 0 0 0 1 1 1 1
  spline S1386 degree 3 poles (-17.8359, 25.1469) (-17.8359, 25.0699) (-17.6891, 24.9145) (-17.6164, 24.9145) knots 0 0 0 0 1 1 1 1
  spline S1387 degree 3 poles (-17.6164, 24.9145) (-17.588, 24.9145) (-17.328, 25.0057) (-17.0386, 25.1171) knots 0 0 0 0 1 1 1 1
  spline S1388 degree 3 poles (-8.2248, 25.2485) (-8.1631, 25.3167) (-7.9872, 25.7183) (-7.834, 26.1411) knots 0 0 0 0 1 1 1 1
  spline S1389 degree 3 poles (-7.834, 26.1411) (-7.1355, 28.0676) (-6.1727, 30.0939) (-5.3796, 31.3067) knots 0 0 0 0 1 1 1 1
  spline S1390 degree 3 poles (-5.3796, 31.3067) (-4.9683, 31.9356) (-4.897, 32.0864) (-4.9574, 32.1992) knots 0 0 0 0 1 1 1 1
  spline S1391 degree 3 poles (-4.9574, 32.1992) (-5.0151, 32.3071) (-5.1055, 32.335) (-5.3978, 32.335) knots 0 0 0 0 1 1 1 1
  spline S1392 degree 3 poles (-5.3978, 32.335) (-5.7566, 32.335) (-5.7808, 32.3217) (-6.3929, 31.7877) knots 0 0 0 0 1 1 1 1
  spline S1393 degree 3 poles (-6.3929, 31.7877) (-7.9392, 30.4389) (-9.4546, 28.5027) (-10.7286, 26.2481) knots 0 0 0 0 1 1 1 1
  spline S1394 degree 3 poles (-10.7286, 26.2481) (-11.063, 25.6562) (-11.0331, 25.5489) (-10.4696, 25.318) knots 0 0 0 0 1 1 1 1
  spline S1395 degree 3 poles (-10.4696, 25.318) (-10.0861, 25.1609) (-9.9231, 25.1372) (-9.1837, 25.1313) knots 0 0 0 0 1 1 1 1
  spline S1396 degree 3 poles (-9.1837, 25.1313) (-8.457, 25.1255) (-8.3211, 25.1421) (-8.2248, 25.2485) knots 0 0 0 0 1 1 1 1
  spline S1397 degree 3 poles (10.1347, 25.2901) (10.1808, 25.4737) (9.548, 26.7968) (8.9089, 27.8533) knots 0 0 0 0 1 1 1 1
  line L170 (8.9089, 27.8533) -> (8.5498, 28.4469)
  line L171 (8.5498, 28.4469) -> (8.7235, 28.7633)
  line L172 (8.7235, 28.7633) -> (8.8972, 29.0798)
  line L173 (8.8972, 29.0798) -> (9.3372, 29.101)
  spline S1398 degree 3 poles (9.3372, 29.101) (10.0884, 29.1373) (10.0727, 29.3059) (9.2377, 30.167) knots 0 0 0 0 1 1 1 1
  spline S1399 degree 3 poles (9.2377, 30.167) (8.0159, 31.4269) (7.0777, 32.1881) (6.6426, 32.2723) knots 0 0 0 0 1 1 1 1
  spline S1400 degree 3 poles (6.6426, 32.2723) (6.1011, 32.3772) (5.8575, 32.3505) (5.7641, 32.176) knots 0 0 0 0 1 1 1 1
  spline S1401 degree 3 poles (5.7641, 32.176) (5.692, 32.0413) (5.7074, 31.9531) (5.8645, 31.5985) knots 0 0 0 0 1 1 1 1
  spline S1402 degree 3 poles (5.8645, 31.5985) (5.9665, 31.3683) (6.1121, 31.0141) (6.1881, 30.8115) knots 0 0 0 0 1 1 1 1
  line L174 (6.1881, 30.8115) -> (6.3263, 30.443)
  line L175 (6.3263, 30.443) -> (6.1122, 30.1518)
  line L176 (6.1122, 30.1518) -> (5.898, 29.8606)
  line L177 (5.898, 29.8606) -> (5.107, 29.8776)
  spline S1403 degree 3 poles (5.107, 29.8776) (4.0411, 29.9005) (4.0667, 29.9324) (4.1877, 28.7297) knots 0 0 0 0 1 1 1 1
  spline S1404 degree 3 poles (4.1877, 28.7297) (4.2381, 28.2292) (4.3303, 27.2842) (4.3926, 26.6296) knots 0 0 0 0 1 1 1 1
  spline S1405 degree 3 poles (4.3926, 26.6296) (4.4649, 25.8703) (4.5403, 25.4015) (4.6007, 25.3345) knots 0 0 0 0 1 1 1 1
  spline S1406 degree 3 poles (4.6007, 25.3345) (4.6793, 25.2475) (5.011, 25.2254) (6.5381, 25.2052) knots 0 0 0 0 1 1 1 1
  spline S1407 degree 3 poles (6.5381, 25.2052) (7.5515, 25.1918) (8.3938, 25.1682) (8.4099, 25.1527) knots 0 0 0 0 1 1 1 1
  spline S1408 degree 3 poles (8.4099, 25.1527) (8.4259, 25.1372) (8.8112, 25.1245) (9.2661, 25.1245) knots 0 0 0 0 1 1 1 1
  spline S1409 degree 3 poles (9.2661, 25.1245) (10.0773, 25.1245) (10.0939, 25.1277) (10.1347, 25.2901) knots 0 0 0 0 1 1 1 1
  spline S1410 degree 3 poles (3.6458, 25.3698) (3.7263, 25.4462) (3.7227, 25.6692) (3.6228, 26.7979) knots 0 0 0 0 1 1 1 1
  spline S1411 degree 3 poles (3.6228, 26.7979) (3.3689, 29.6658) (3.3244, 29.8848) (2.9955, 29.8848) knots 0 0 0 0 1 1 1 1
  spline S1412 degree 3 poles (2.9955, 29.8848) (2.9115, 29.8848) (2.7432, 29.9876) (2.6215, 30.1132) knots 0 0 0 0 1 1 1 1
  spline S1413 degree 3 poles (2.6215, 30.1132) (2.4197, 30.3214) (2.3852, 30.4271) (2.2307, 31.3103) knots 0 0 0 0 1 1 1 1
  spline S1414 degree 3 poles (2.2307, 31.3103) (2.1215, 31.9345) (2.0201, 32.32) (1.9453, 32.3945) knots 0 0 0 0 1 1 1 1
  spline S1415 degree 3 poles (1.9453, 32.3945) (1.841, 32.4984) (1.5647, 32.5081) (-0.8103, 32.4915) knots 0 0 0 0 1 1 1 1
  spline S1416 degree 3 poles (-0.8103, 32.4915) (-3.8425, 32.4703) (-3.5628, 32.5334) (-4.1652, 31.7343) knots 0 0 0 0 1 1 1 1
  spline S1417 degree 3 poles (-4.1652, 31.7343) (-5.0394, 30.5747) (-5.9671, 28.8093) (-6.8067, 26.7075) knots 0 0 0 0 1 1 1 1
  spline S1418 degree 3 poles (-6.8067, 26.7075) (-7.1904, 25.747) (-7.2658, 25.4964) (-7.2088, 25.3713) knots 0 0 0 0 1 1 1 1
  line L178 (-7.2088, 25.3713) -> (-7.1386, 25.2172)
  line L179 (-7.1386, 25.2172) -> (-1.7941, 25.2482)
  spline S1419 degree 3 poles (-1.7941, 25.2482) (2.4483, 25.2728) (3.5701, 25.2979) (3.6458, 25.3698) knots 0 0 0 0 1 1 1 1
  spline S1420 degree 3 poles (14.7021, 25.9786) (14.8413, 26.1178) (14.7982, 26.2756) (14.5586, 26.5039) knots 0 0 0 0 1 1 1 1
  spline S1421 degree 3 poles (14.5586, 26.5039) (14.3447, 26.7076) (14.2827, 26.7252) (13.526, 26.7966) knots 0 0 0 0 1 1 1 1
  spline S1422 degree 3 poles (13.526, 26.7966) (13.0832, 26.8384) (12.2266, 26.8936) (11.6224, 26.9193) knots 0 0 0 0 1 1 1 1
  line L180 (11.6224, 26.9193) -> (10.5239, 26.966)
  line L181 (10.5239, 26.966) -> (10.4792, 26.7879)
  spline S1423 degree 3 poles (10.4792, 26.7879) (10.4255, 26.5741) (10.6001, 26.2002) (10.7776, 26.1488) knots 0 0 0 0 1 1 1 1
  spline S1424 degree 3 poles (10.7776, 26.1488) (10.8454, 26.1291) (11.6096, 26.0761) (12.476, 26.0309) knots 0 0 0 0 1 1 1 1
  spline S1425 degree 3 poles (12.476, 26.0309) (13.3423, 25.9858) (14.0642, 25.9366) (14.0802, 25.9217) knots 0 0 0 0 1 1 1 1
  spline S1426 degree 3 poles (14.0802, 25.9217) (14.1486, 25.8581) (14.6252, 25.9017) (14.7021, 25.9786) knots 0 0 0 0 1 1 1 1
  spline S1427 degree 3 poles (13.3581, 27.753) (13.3957, 27.9029) (13.3373, 28.0005) (12.9919, 28.3655) knots 0 0 0 0 1 1 1 1
  spline S1428 degree 3 poles (12.9919, 28.3655) (12.149, 29.2562) (11.8912, 29.4613) (11.5569, 29.5071) knots 0 0 0 0 1 1 1 1
  spline S1429 degree 3 poles (11.5569, 29.5071) (11.2734, 29.5459) (11.238, 29.5341) (11.1663, 29.3766) knots 0 0 0 0 1 1 1 1
  spline S1430 degree 3 poles (11.1663, 29.3766) (11.1033, 29.2385) (11.1086, 29.182) (11.1924, 29.0982) knots 0 0 0 0 1 1 1 1
  spline S1431 degree 3 poles (11.1924, 29.0982) (11.2859, 29.0047) (11.2771, 28.9527) (11.1127, 28.6283) knots 0 0 0 0 1 1 1 1
  line L182 (11.1127, 28.6283) -> (10.9278, 28.2635)
  line L183 (10.9278, 28.2635) -> (10.4237, 28.3108)
  spline S1432 degree 3 poles (10.4237, 28.3108) (9.9774, 28.3526) (9.9053, 28.3423) (9.796, 28.2215) knots 0 0 0 0 1 1 1 1
  spline S1433 degree 3 poles (9.796, 28.2215) (9.6442, 28.0538) (9.7027, 27.8676) (9.9349, 27.7793) knots 0 0 0 0 1 1 1 1
  spline S1434 degree 3 poles (9.9349, 27.7793) (10.0284, 27.7438) (10.3943, 27.7113) (10.7479, 27.7073) knots 0 0 0 0 1 1 1 1
  spline S1435 degree 3 poles (10.7479, 27.7073) (11.1015, 27.7032) (11.6744, 27.6767) (12.0209, 27.6484) knots 0 0 0 0 1 1 1 1
  spline S1436 degree 3 poles (12.0209, 27.6484) (13.2507, 27.5478) (13.3077, 27.5523) (13.3581, 27.753) knots 0 0 0 0 1 1 1 1
  spline S1437 degree 3 poles (5.2196, 30.7159) (5.2834, 30.7688) (5.3355, 30.8438) (5.3355, 30.8826) knots 0 0 0 0 1 1 1 1
  spline S1438 degree 3 poles (5.3355, 30.8826) (5.3355, 31.003) (4.7681, 32.254) (4.6805, 32.3267) knots 0 0 0 0 1 1 1 1
  spline S1439 degree 3 poles (4.6805, 32.3267) (4.6349, 32.3645) (4.2518, 32.4171) (3.829, 32.4436) knots 0 0 0 0 1 1 1 1
  spline S1440 degree 3 poles (3.829, 32.4436) (3.1267, 32.4876) (3.05, 32.4802) (2.9406, 32.3584) knots 0 0 0 0 1 1 1 1
  spline S1441 degree 3 poles (2.9406, 32.3584) (2.8294, 32.2345) (2.8285, 32.1827) (2.9277, 31.6325) knots 0 0 0 0 1 1 1 1
  spline S1442 degree 3 poles (2.9277, 31.6325) (3.0985, 30.6843) (3.0872, 30.6961) (3.8678, 30.6549) knots 0 0 0 0 1 1 1 1
  spline S1443 degree 3 poles (3.8678, 30.6549) (4.8763, 30.6016) (5.0935, 30.6114) (5.2196, 30.7159) knots 0 0 0 0 1 1 1 1
  spline S1444 degree 3 poles (-9.1554, 32.784) (-8.6135, 32.8691) (-5.3848, 33.1088) (-3.9051, 33.1739) knots 0 0 0 0 1 1 1 1
  spline S1445 degree 3 poles (-3.9051, 33.1739) (-3.0388, 33.212) (-1.1104, 33.2436) (0.3802, 33.2441) knots 0 0 0 0 1 1 1 1
  spline S1446 degree 3 poles (0.3802, 33.2441) (2.9853, 33.2449) (3.0933, 33.2503) (3.1627, 33.3801) knots 0 0 0 0 1 1 1 1
  spline S1447 degree 3 poles (3.1627, 33.3801) (3.2552, 33.5529) (3.0669, 33.7089) (2.3715, 34.0356) knots 0 0 0 0 1 1 1 1
  spline S1448 degree 3 poles (2.3715, 34.0356) (1.399, 34.4925) (1.1226, 34.5405) (-0.5099, 34.5362) knots 0 0 0 0 1 1 1 1
  spline S1449 degree 3 poles (-0.5099, 34.5362) (-3.2169, 34.529) (-6.2004, 34.1005) (-9.0679, 33.307) knots 0 0 0 0 1 1 1 1
  spline S1450 degree 3 poles (-9.0679, 33.307) (-9.7693, 33.1129) (-9.8554, 33.0721) (-9.8554, 32.9337) knots 0 0 0 0 1 1 1 1
  spline S1451 degree 3 poles (-9.8554, 32.9337) (-9.8554, 32.725) (-9.7913, 32.6738) (-9.5788, 32.7128) knots 0 0 0 0 1 1 1 1
  spline S1452 degree 3 poles (-9.5788, 32.7128) (-9.4807, 32.7308) (-9.2901, 32.7629) (-9.1554, 32.784) knots 0 0 0 0 1 1 1 1
  line L184 (42.5, -42.5) -> (-42.5, -42.5)
  line L185 (-42.5, -42.5) -> (-42.5, 42.5)
  line L186 (-42.5, 42.5) -> (42.5, 42.5)
  line L187 (42.5, 42.5) -> (42.5, -42.5)
  line L188 (42.5, -42.5) -> (-42.5, 42.5) construction
  line L189 (-42.5, -42.5) -> (42.5, 42.5) construction
  dimension "d1" = 85
  dimension "d2" = 85
  constraint horizontal L184
  constraint perpendicular L184 L185
  constraint parallel L184 L186
  constraint parallel L185 L187
  constraint coincident L188 origin
  constraint coincident L189 origin
  measures "d1" distance of L185.end L186.end
  measures "d2" distance of L184.end L185.end